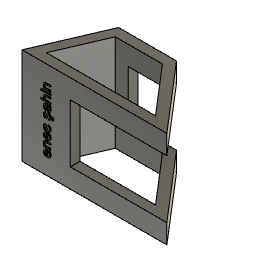
Model 27 (Autodesk Fusion 360 design; units mm, degrees)
Autodesk Fusion 360 part; units mm, degrees
sketch "Sketch1" plane through (0, 0, 0) normal (0, 0, 1) x (1, 0, 0)
  line L0 (15, 35) -> (-45, 35)
  line L1 (-75, 35) -> (-75, -35) construction
  line L2 (-75, -35) -> (75, -35)
  line L3 (75, -35) -> (75, 35) construction
  line L4 (75, 35) -> (-75, -35) construction
  line L5 (-75, 35) -> (75, -35) construction
  line L6 (75, 35) -> (15, 35) construction
  line L7 (15, 35) -> (-45, 35) construction
  line L8 (15, 35) -> (75, -35)
  line L9 (-45, 35) -> (-75, -35)
  line L10 (-45, 35) -> (-75, 35) construction
  line L11 (10.4007, 25) -> (53.2578, -25)
  line L12 (-59.8346, -25) -> (53.2578, -25)
  line L13 (-38.406, 25) -> (-59.8346, -25)
  line L14 (10.4007, 25) -> (-38.406, 25)
  dimension "d1" = 150
  dimension "d2" = 70
  dimension "d3" = 60
  dimension "d4" = 60
  dimension "d5" = -10
  constraint horizontal L0
  constraint perpendicular L0 L1
  constraint parallel L0 L2
  constraint parallel L1 L3
  constraint coincident L4 origin
  constraint coincident L5 origin
  constraint perpendicular L3 L6
  constraint parallel L0 L7
  measures "d1" distance of L1.end L2.end
  measures "d2" distance of L1.start L1.end
  measures "d3" distance of L3.end L0.start
  measures "d4" distance of L0.start L0.end
extrude "Extrude1" add sketch "Sketch1" along normal blind 100
sketch "Sketch3" plane through (0, 35, 0) normal (0, 1, 0) x (-1, 0, 0)
  line L0 (-15, 0) -> (45, 0)
  line L1 (45, 0) -> (45, 100)
  line L2 (45, 100) -> (-15, 100)
  line L3 (-15, 100) -> (-15, 0)
  line L4 (75, 100) -> (25, 100) construction
  line L5 (75, 100) -> (75, 0) construction
  line L6 (75, 0) -> (25, 0) construction
  line L7 (25, 100) -> (25, 80) construction
  line L8 (25, 0) -> (25, 20) construction
  line L9 (25, 80) -> (-90, 80)
  line L10 (25, 20) -> (-90, 20)
  line L11 (-90, 20) -> (-90, 80)
  line L12 (25, 80) -> (25, 20)
  dimension "d8" = 50
  dimension "d9" = 50
  dimension "d10" = 100
  dimension "d11" = 20
  dimension "d12" = 20
  constraint horizontal L4
  constraint perpendicular L4 L5
  constraint perpendicular L5 L6
  constraint perpendicular L4 L7
  constraint perpendicular L6 L8
  constraint perpendicular L3 L9
  constraint perpendicular L8 L10
  constraint perpendicular L9 L11
  measures "d8" distance of L4.start L4.end
  measures "d9" distance of L5.end L6.end
  measures "d10" distance of L4.end L6.end
  measures "d11" distance of L4.end L7.end
  measures "d12" distance of L6.end L8.end
extrude "Extrude2" cut sketch "Sketch3" against normal blind 70 contours L3 L9 L10 L11 | L3 L9 L10 L12
ref_plane "WorkPlane1" through (0, -35, 50) normal (0, -1, 0) x (1, 0, 0)
sketch "Sketch4" plane through (0, -35, 50) normal (0, -1, 0) x (1, 0, 0)
  line L0 (-30, -40) -> (-30, 40) construction
  line L1 (-30, 40) -> (-70, 40) construction
  line L2 (-70, 40) -> (-70, -40) construction
  line L3 (-70, -40) -> (-30, -40) construction
  text T0 "enes şahin" font "Arial" height 10 align centre middle in box 80 x 40 at (-30, -40) x (0, 1) y (-1, 0) spacing 1
extrude "Extrude3" add sketch "Sketch4" along normal blind 0.5 text T0
